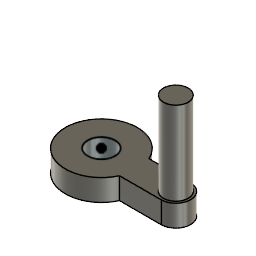
Grank (Autodesk Fusion 360 design; units mm, degrees)
Autodesk Fusion 360 part; units mm, degrees
sketch "Sketch5" plane through (0, 0, 0) normal (0, 0, 1) x (1, 0, 0)
  line L0 (9.3481, 1.8494) -> (4.1024, 1.8494)
  line L1 (9.3481, -1.8494) -> (4.1024, -1.8494)
  arc A0 (9.2519, -1.8494) -> (9.2519, 1.8494) centre (9.3, 0) ccw
  arc A1 (4.1024, 1.8494) -> (4.1024, -1.8494) centre (0, 0) ccw
  dimension "d23" = 9
  dimension "d24" = 3.7
  dimension "d25" = 9.3
  constraint coincident A1.centre origin
  constraint coincident L0.start A0
  constraint horizontal L0
  constraint coincident L1.start A0
  constraint parallel L0 L1
  constraint coincident L0 A0.end
  constraint coincident L1 A0.start
  measures "d23" diameter of A1
  measures "d24" diameter of A0
  measures "d25" distance of A1.centre A0.centre
sketch "Sketch6" plane through (0, 0, 0) normal (0, 0, 1) x (1, 0, 0)
  circle A0 centre (0, 0) radius 1.7
  dimension "d26" = 3.4
  constraint coincident A0.centre origin
  measures "d26" diameter of A0
extrude "Extrude6" add sketch "Sketch5" against normal blind 2.7
hole "Hole2" at (0, 0, 0) direction (0, 0, -1) diameter 3.4 depth 2.7 tip angle 118
sketch "Sketch7" plane through (0, 0, 0) normal (0, 0, 1) x (1, 0, 0)
  circle A0 centre (9.3, 0) radius 1.55
  dimension "d32" = 3.1
  dimension "d33" = 9.3
  measures "d32" diameter of A0
  measures "d33" distance of A0.centre origin
extrude "Extrude7" add sketch "Sketch7" along normal blind 10.4
sketch "Sketch1" plane through (0, 0, 0) normal (0, 0, 1) x (1, 0, 0)
  circle A0 centre (0, 0) radius 10.7065
  dimension "d1" = 21.413
  constraint coincident A0.centre origin
  measures "d1" diameter of A0
extrude "Extrude1" [suppressed]
sketch "Sketch2" plane through (0, 0, 0) normal (0, 0, 1) x (1, 0, 0)
  circle A0 centre (0, 0) radius 1.5
  dimension "d4" = 3
  constraint coincident A0.centre origin
  measures "d4" diameter of A0
sketch "Sketch3" plane through (0, 0, 0) normal (0, 0, 1) x (1, 0, 0)
  circle A0 centre (0, 0) radius 1.5
  circle A1 centre (7.5, 0) radius 1.5
  dimension "d7" = 3
  dimension "d9" = 3
  dimension "d10" = 7.5
  constraint coincident A0.centre origin
  measures "d7" diameter of A0
  measures "d9" diameter of A1
  measures "d10" distance of A0.centre A1.centre
sketch "Sketch4" plane through (0, 0, 0) normal (0, 0, 1) x (1, 0, 0)
  circle A0 centre (0, 0) radius 1.5
  dimension "d8" = 3
  constraint coincident A0.centre origin
  measures "d8" diameter of A0
extrude "Extrude3" [suppressed]
hole "Hole1" [suppressed]
extrude "Extrude4" [suppressed]
extrude "Extrude5" [suppressed]
split "Split1" [suppressed]
